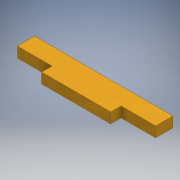
# Autodesk Inventor part: Celda riel
Saved by Autodesk Inventor 2018 (Build 220112000, 112)
## iProperties
Created: 2020-03-13
Part Number: Celda riel
Material: Genérico
Document SubType Name: Modeling
Designer: joser
Density: 1 g/cm^3
Appearance: Soldadura - Latón
Author: joser
Autodesk Inventor part; units mm, degrees
ref_plane "YZ Plane" through (0, 0, 0) normal (1, 0, 0) x (0, 1, 0)
ref_plane "XZ Plane" through (0, 0, 0) normal (0, 1, 0) x (-1, 0, 0)
ref_plane "XY Plane" through (0, 0, 0) normal (0, 0, 1) x (1, 0, 0)
sketch "Boceto1" plane through (0, 0, 0) normal (0, 0, 1) x (1, 0, 0)
  line L0 (0, 5) -> (40, 5)
  line L1 (40, 5) -> (40, 0)
  line L2 (0, 0) -> (0, 5)
  line L3 (10, 0) -> (10, -3)
  line L4 (10, -3) -> (30, -3)
  line L5 (30, -3) -> (30, 0)
  line L6 (40, 0) -> (30, 0)
  line L7 (10, 0) -> (0, 0)
  dimension "d2" = 40
  dimension "d4" = 20
  dimension "d6" = 3
  dimension "d7" = 5
  dimension "d8" = 10
  constraints: 16 end point, 3 parallel, 3 perpendicular, 1 coincident, 1 collinear, 1 horizontal, 1 vertical
  measures "d2" distance between parallel lines of L1 L2
  measures "d4" distance of L3.end L4.end
  measures "d6" distance between parallel lines of L7 L4
  measures "d7" distance between parallel lines of L0 L6
  measures "d8" distance between parallel lines of L2 L3
extrude "Extrusión1" add sketch "Boceto1" along normal blind 3
